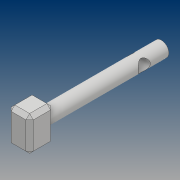
# Autodesk Inventor part: 槌子
Saved by Autodesk Inventor 2018 (Build 220112000, 112)
## iProperties
Created: 2020-11-30
Part Number: 槌子
Material: 一般
Document SubType Name: Modeling
Designer: 88697
Density: 1 g/cm^3
Appearance: 預設
Author: 88697
Autodesk Inventor part; units mm, degrees
ref_plane "YZ Plane" through (0, 0, 0) normal (1, 0, 0) x (0, 1, 0)
ref_plane "XZ Plane" through (0, 0, 0) normal (0, 1, 0) x (-1, 0, 0)
sketch "草圖1" plane through (0, 0, 0) normal (0, 0, 1) x (1, 0, 0)
  line L0 (0, 0) -> (3, 0)
  line L1 (3, 0) -> (3, 58)
  line L2 (3, 58) -> (0, 58)
  line L3 (0, 58) -> (0, 0)
  dimension "d0" = 58
  dimension "d1" = 3
  constraints: 8 end point, 2 parallel, 1 horizontal, 1 perpendicular
  measures "d0" distance of L0.end L1.end
  measures "d1" distance between parallel lines of L3 L1
revolve "迴轉1" add sketch "草圖1" angle 360 about axis through (0, 58, 0) along (0, -1, 0)
ref_plane "工作平面1" through (0, 48, 0) normal (0, 1, 0) x (1, 0, 0)
sketch "草圖2" plane through (0, 48, 0) normal (0, 1, 0) x (1, 0, 0)
  line L0 (-10.3022, 0) -> (10.735, 0)
  line L1 (10.735, 0) -> (10.735, 2.5)
  line L2 (10.735, 2.5) -> (-10.3022, 2.5)
  line L3 (-10.3022, 2.5) -> (-10.3022, 0)
  point P0 (0, 0)
  dimension "d4" = 2.5
  dimension "d5" = 0
  constraints: 8 end point, 2 parallel, 1 horizontal, 1 perpendicular
  measures "d4" distance of L0.end L1.end
  measures "d5" distance from line of point (0, 0) L0
revolve "迴轉2" cut sketch "草圖2" angle 360 about axis through (-10.3022, 48, 0) along (1, 0, 0)
sketch "草圖3" plane through (0, 0, 0) normal (0, -1, 0) x (1, 0, 0)
  line L0 (-4.5, 7) -> (4.5, 7)
  line L1 (4.5, 7) -> (4.5, -7)
  line L2 (4.5, -7) -> (-4.5, -7)
  line L3 (-4.5, -7) -> (-4.5, 7)
  point P0 (0, 0)
  dimension "d7" = 9
  dimension "d8" = 4.5
  dimension "d9" = 14
  dimension "d10" = 7
  constraints: 8 end point, 2 parallel, 1 horizontal, 1 perpendicular
  measures "d7" distance of L1.end L2.end
  measures "d8" distance from line of L1 point (0, 0)
  measures "d9" distance between parallel lines of L2 L0
  measures "d10" distance from line of point (0, 0) L0
extrude "擠出1" add sketch "草圖3" against normal blind 10
chamfer "倒角1" distance 1.5 angle 45 12 edges at (4.5, 5, -7) (4.5, 5, 7) (-4.5, 5, 7) (-4.5, 5, -7) (0, 0, -7) (-4.5, 0, 0) (4.5, 0, 0) (0, 0, 7) (0, 10, -7) (4.5, 10, 0) (0, 10, 7) (-4.5, 10, 0)
